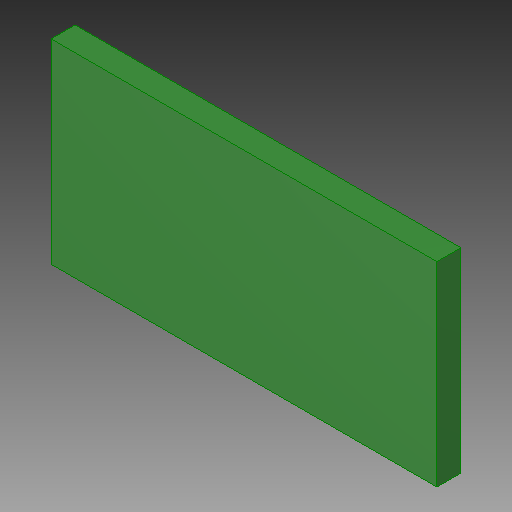
# Autodesk Inventor part: XT60
Saved by Autodesk Inventor 2017 (Build 210142000, 142)
## iProperties
Created: 2019-06-13
Part Number: XT60
Material: Generic
Document SubType Name: Modeling
Designer: Marc
Density: 1 g/cm^3
Appearance: XT60, XT60
Author: Marc
Autodesk Inventor part; units mm, degrees
ref_plane "YZ Plane" through (0, 0, 0) normal (1, 0, 0) x (0, 1, 0)
ref_plane "XZ Plane" through (0, 0, 0) normal (0, 1, 0) x (-1, 0, 0)
ref_plane "XY Plane" through (0, 0, 0) normal (0, 0, 1) x (1, 0, 0)
sketch "XT60, XT60_61" plane through (0, 0, 0) normal (0, 0, 1) x (1, 0, 0)
  line L0 (-8.0635, 4.0635) -> (8, 4.0635)
  line L1 (8, 4.0635) -> (8, -4.0635)
  line L2 (8, -4.0635) -> (-8.0635, -4.0635)
  line L3 (-8.0635, -4.0635) -> (-8.0635, 4.0635)
  constraints: 8 end point
extrude "Extrusion1" add sketch "XT60, XT60_61" along normal blind 1
body "Solid1"
